Autodesk Fusion 360 part; units mm, degrees
(part 2 of 2)
  constraint parallel L239 L241
  constraint parallel L240 L242
  constraint tangent L240 A253
  constraint tangent A253 L241
  constraint tangent A254 L242
  constraint tangent L241 A254
  constraint tangent L237 A250
  constraint tangent A250 L238
  constraint tangent L238 A251
  constraint tangent L242 A255
  constraint tangent L239 A255
  constraint tangent L239 A252
  constraint tangent A252 L240
  constraint horizontal L243
  constraint perpendicular L243 L244
  constraint parallel L243 L245
  constraint parallel L244 L246
  constraint tangent A259 L246
  constraint tangent L245 A259
  constraint tangent L244 A258
  constraint tangent A258 L245
  constraint tangent A257 L244
  constraint tangent L243 A257
  constraint tangent A256 L243
  constraint tangent A256 L246
  constraint tangent L247 A260
  constraint tangent L249 A260
  constraint tangent L248 A261
  constraint tangent L249 A261
  constraint tangent L205 A262
  constraint tangent L250 A262
  constraint tangent L206 A263
  constraint tangent L250 A263
  constraint tangent L218 A264
  constraint tangent L251 A264
  constraint tangent L219 A265
  constraint tangent L251 A265
  constraint tangent L195 A266
  constraint tangent L252 A266
  constraint tangent L194 A267
  constraint tangent L252 A267
  constraint tangent L109 A268
  measures "d1" diameter of A0
  measures "d2" diameter of A1
  measures "d3" diameter of A2
  measures "d4" diameter of A3
  measures "d5" diameter of A4
  measures "d9" diameter of A110
  measures "d12" diameter of A111
  measures "d318" diameter of A181
  measures "d319" diameter of A182
extrude "Extrude1" add sketch "mriya-bumper-mjf" along normal blind 10.5 contours L106 L107 L147 A142 L148 L164 L165 A158 | L106 L107 L138 A133 L139 A134 L140 A135 L141 A136 L142 A137 L143 A138 L144 A139 L145 A140 L146 A141 L147 L148 A143 L149 A144 L150 A145 L151 A146 L152 A147 L153 A148 L154 A149 L155 A150 L156 A151 L157 A152 L158 A153 L159 A154 L160 L161 L162 L163 L164 L165 L166 L167 L168 L169 L170 L171 L172 L173 L174 A155 A156 A157 A159 A160 A161 A162 A163 L180 L181 L182 L183 L184 L185 L186 A168 A169 A170 A171 A172 A173 A174 A175 A176 A177 A178 A179 A180 makes body 1
extrude "Extrude2" add sketch "mriya-bumper-mjf" along normal blind 17 contours L106 L107 L147 A142 L148 L164 L165 A158 bodies 1
extrude "Extrude3" add sketch "mriya-bumper-mjf" along normal blind 2 from surface at 1.7 contours L108 L109 L110 L138 A133 L139 A134 L140 A135 L141 A136 L142 A137 L143 A138 L144 A139 L145 A140 L146 A141 L147 L148 A143 L149 A144 L150 A145 L151 A146 L152 A147 L153 A148 L154 A149 L155 A150 L156 A151 L157 A152 L158 A153 L159 A154 A183 A184 A185 A186 A268 | L110 L148 A183 A184 | L108 L109 L147 A142 L148 A185 A186 A268 | A113 | A114 | A115 | A116 | A181 | A182 bodies 1
extrude "Extrude6" add sketch "mriya-bumper-mjf" along normal blind 1 from surface at 14.3 contours L108 L109 L147 A142 L148 A185 A186 A268 bodies 1
extrude "Extrude13" add sketch "mriya-bumper-mjf" along normal blind 1 from surface at 7.7 contours L110 L148 A183 A184 bodies 1
chamfer "Chamfer7" distance 0.599 angle 45 4 edges at (-7, 58.2432, 14.3) (-7.4686, 77.6246, 14.3) (-14.85, 78.0932, 14.3) (-7, 9.5932, 7.7) on bodies 1
sketch "power-switch" plane through (-4.5, 0, 0) normal (1, 0, 0) x (0, 1, 0)
  line L0 (1.9932, 0) -> (76.4932, 0)
  line L1 (76.4932, 0) -> (76.4932, 17)
  line L2 (76.4932, 17) -> (19.2932, 17)
  line L3 (19.2932, 17) -> (19.2932, 10.5)
  line L4 (19.2932, 10.5) -> (1.9932, 10.5)
  line L5 (1.9932, 10.5) -> (1.9932, 0)
  line L6 (35.9932, 5.2) -> (25.7932, 5.2)
  line L7 (25.7932, 5.2) -> (25.7932, 7.9)
  line L8 (25.7932, 7.9) -> (35.9932, 7.9)
  line L9 (35.9932, 7.9) -> (35.9932, 5.2)
  line L10 (37.3932, 2.8) -> (24.3932, 2.8)
  line L11 (23.3932, 3.8) -> (23.3932, 9.3)
  line L12 (24.3932, 10.3) -> (37.3932, 10.3)
  line L13 (38.3932, 9.3) -> (38.3932, 3.8)
  arc A0 (24.3932, 10.3) -> (23.3932, 9.3) centre (24.3932, 9.3) ccw
  arc A1 (38.3932, 9.3) -> (37.3932, 10.3) centre (37.3932, 9.3) ccw
  arc A2 (37.3932, 2.8) -> (38.3932, 3.8) centre (37.3932, 3.8) ccw
  arc A3 (23.3932, 3.8) -> (24.3932, 2.8) centre (24.3932, 3.8) ccw
  line L14 (19.2932, 10.5) -> (1.8932, 10.5)
  line L15 (1.8932, 10.5) -> (1.8932, 0)
  line L16 (1.8932, 0) -> (76.5932, 0)
  line L17 (76.5932, 0) -> (76.5932, 17)
  line L18 (76.5932, 17) -> (19.2932, 17)
  line L19 (19.2932, 17) -> (19.2932, 10.5)
  constraint perpendicular L6 L7
  constraint tangent L11 A0
  constraint tangent L12 A0
  constraint tangent L12 A1
  constraint tangent L13 A1
  constraint tangent L10 A2
  constraint tangent L13 A2
  constraint tangent L10 A3
  constraint tangent L11 A3
  constraint vertical L7
  constraint perpendicular L7 L8
  constraint vertical L9
extrude "Extrude8" cut sketch "power-switch" against normal blind 2.5 contours L6 L7 L8 L9 bodies 1
extrude "Extrude9" cut sketch "power-switch" against normal blind 1 contours L10 L11 L12 L13 A0 A1 A2 A3 bodies 1
fillet "Fillet23" radius 0.1 8 edges at (-4.5, 23.3932, 6.55) (-4.5, 23.6861, 10.0071) (-4.5, 30.8932, 10.3) (-4.5, 38.1003, 10.0071) (-4.5, 38.3932, 6.55) (-4.5, 38.1003, 3.0929) (-4.5, 30.8932, 2.8) (-4.5, 23.6861, 3.0929) on bodies 1
fillet "Fillet24" radius 1 8 edges at (-5.5, 30.8932, 2.8) (-5.5, 23.6861, 3.0929) (-5.5, 23.3932, 6.55) (-5.5, 23.6861, 10.0071) (-5.5, 30.8932, 10.3) (-5.5, 38.1003, 10.0071) (-5.5, 38.3932, 6.55) (-5.5, 38.1003, 3.0929) on bodies 1
chamfer "Chamfer4" distance 0.5 angle 45 4 edges at (-7, 30.8932, 5.2) (-7, 35.9932, 6.55) (-7, 30.8932, 7.9) (-7, 25.7932, 6.55) on bodies 1
sketch "usb-c" plane through (0, 80.5932, 0) normal (0, 1, 0) x (-1, 0, 0)
  line L0 (8.5, 0) -> (40.9017, 0)
  line L1 (40.9017, 0) -> (40.9017, 10.5)
  line L2 (40.9017, 10.5) -> (25.8, 10.5)
  line L3 (25.8, 10.5) -> (25.8, 17)
  line L4 (25.8, 17) -> (8.5, 17)
  line L5 (8.5, 17) -> (8.5, 0)
  line L6 (19.7003, 7) -> (13.1002, 7)
  line L7 (13.1002, 12.35) -> (19.7002, 12.35)
  line L8 (19.7002, 8.85) -> (13.1002, 8.85)
  line L9 (21.0002, 11.05) -> (21.0002, 10.15)
  line L10 (13.1002, 14.2) -> (19.7003, 14.2)
  line L11 (11.8003, 10.15) -> (11.8003, 11.05)
  arc A0 (13.1002, 12.35) -> (11.8003, 11.05) centre (13.1002, 11.05) ccw
  arc A1 (11.8003, 10.15) -> (13.1003, 8.85) centre (13.1002, 10.15) ccw
  arc A2 (21.0002, 11.05) -> (19.7002, 12.35) centre (19.7002, 11.05) ccw
  arc A3 (19.7002, 8.85) -> (21.0002, 10.15) centre (19.7003, 10.15) ccw
  line L12 (22.7003, 11.2) -> (22.7003, 10)
  line L13 (10.1002, 11.2) -> (10.1002, 10)
  arc A4 (22.7002, 11.2) -> (19.7003, 14.2) centre (19.7003, 11.2) ccw
  arc A5 (19.7003, 7) -> (22.7003, 10) centre (19.7003, 10) ccw
  arc A6 (13.1002, 14.2) -> (10.1002, 11.2) centre (13.1002, 11.2) ccw
  arc A7 (10.1002, 10) -> (13.1002, 7) centre (13.1002, 10) ccw
  dimension "d380" = 3
  dimension "d381" = 3
  dimension "d382" = 3
  dimension "d383" = 3
  constraint horizontal L6
  constraint tangent L11 A0
  constraint tangent L7 A0
  constraint tangent L8 A1
  constraint tangent L11 A1
  constraint tangent L7 A2
  constraint tangent L9 A2
  constraint tangent L9 A3
  constraint tangent L8 A3
  constraint parallel L11 L12
  constraint parallel L5 L13
  constraint tangent L10 A4
  constraint tangent L12 A4
  constraint tangent L12 A5
  constraint tangent L6 A5
  constraint tangent L13 A6
  constraint tangent L10 A6
  constraint tangent L6 A7
  constraint tangent L13 A7
  measures "d380" radius of A4
  measures "d381" radius of A5
  measures "d382" radius of A6
  measures "d383" radius of A7
extrude "Extrude10" cut sketch "usb-c" against normal blind 2.5 contours L7 L8 L9 L11 A0 A1 A2 A3 bodies 1
extrude "Extrude11" cut sketch "usb-c" against normal blind 1.2 contours L6 L10 L12 L13 A4 A5 A6 A7 bodies 1
fillet "Fillet16" radius 1 8 edges at (-16.4003, 79.3932, 7) (-10.9789, 79.3932, 7.8787) (-10.1003, 79.3932, 10.6) (-10.9789, 79.3932, 13.3213) (-16.4003, 79.3932, 14.2) (-21.8216, 79.3932, 13.3213) (-22.7003, 79.3932, 10.6) (-21.8216, 79.3932, 7.8787) on bodies 1
fillet "Fillet20" radius 0.1 8 edges at (-10.9789, 80.5932, 7.8787) (-10.1003, 80.5932, 10.6) (-10.9789, 80.5932, 13.3213) (-16.4003, 80.5932, 14.2) (-21.8216, 80.5932, 13.3213) (-22.7003, 80.5932, 10.6) (-21.8216, 80.5932, 7.8787) (-16.4003, 80.5932, 7) on bodies 1
fillet "Fillet27" radius 1.6 90 edges at (-4.5, 47.9432, 17) (-5.6716, 79.4216, 17) (-17.15, 80.5932, 17) (-33.3509, 80.5932, 10.5) (-41.4757, 80.7074, 10.5) (-42.3069, 81.3771, 10.5) (-43.9492, 82.5887, 10.5) (-51.5908, 82.8932, 10.5) (-58.2758, 83.0074, 10.5) (-60.2069, 84.7771, 10.5) (-62.9492, 87.0887, 10.5) (-73.4, 87.3932, 10.5) (-83.8508, 87.0887, 10.5) (-86.0931, 85.2771, 10.5) (-87.5243, 84.0074, 10.5) (-94.7092, 83.8932, 10.5) (-102.8508, 83.5887, 10.5) (-107.3431, 79.5271, 10.5) (-111.0243, 76.0074, 10.5) (-115.9592, 75.8932, 10.5) (-121.8508, 75.5887, 10.5) (-123.4931, 74.3771, 10.5) (-124.3243, 73.7074, 10.5) (-131.5491, 73.5932, 10.5) (-141.0284, 72.4216, 10.5) (-142.2, 42.8932, 10.5) (-141.0284, 13.3648, 10.5) (-120.4435, 12.1932, 10.5) (-100.9649, 12.5357, 10.5) (-96.4569, 16.5593, 10.5) (-92.76, 20.041, 10.5) (-84.5813, 20.1932, 10.5) (-75.6559, 19.7842, 10.5) (-70.5608, 11.5973, 10.5) (-65.0991, 3.0385, 10.5) (-55.9906, 2.4932, 10.5) (-48.3243, 2.379, 10.5) (-47.4931, 1.7093, 10.5) (-45.8508, 0.4977, 10.5) (-37.1092, 0.1932, 10.5) (-29.3243, 0.079, 10.5) (-28.4931, -0.5907, 10.5) (-26.8508, -1.8023, 10.5) (-16.91, -2.1068, 10.5) (-5.6716, -0.9352, 10.5) (-4.5, 10.5932, 10.5) (-24.7009, 80.5932, 0) (-5.6716, 79.4216, 0) (-4.5, 39.2432, 0) (-5.6716, -0.9352, 0) (-16.91, -2.1068, 0) (-26.8508, -1.8023, 0) (-28.4931, -0.5907, 0) (-29.3243, 0.079, 0) (-37.1092, 0.1932, 0) (-45.8508, 0.4977, 0) (-47.4931, 1.7093, 0) (-48.3243, 2.379, 0) (-55.9906, 2.4932, 0) (-65.0991, 3.0385, 0) (-70.5608, 11.5973, 0) (-75.6559, 19.7842, 0) (-84.5813, 20.1932, 0) (-92.76, 20.041, 0) (-96.4569, 16.5593, 0) (-100.9649, 12.5357, 0) (-120.4435, 12.1932, 0) (-141.0284, 13.3648, 0) (-142.2, 42.8932, 0) (-141.0284, 72.4216, 0) (-131.5491, 73.5932, 0) (-124.3243, 73.7074, 0) (-123.4931, 74.3771, 0) (-121.8508, 75.5887, 0) (-115.9592, 75.8932, 0) (-111.0243, 76.0074, 0) (-107.3431, 79.5271, 0) (-102.8508, 83.5887, 0) (-94.7092, 83.8932, 0) (-87.5243, 84.0074, 0) (-86.0931, 85.2771, 0) (-83.8508, 87.0887, 0) (-73.4, 87.3932, 0) (-62.9492, 87.0887, 0) (-60.2069, 84.7771, 0) (-58.2758, 83.0074, 0) (-51.5908, 82.8932, 0) (-43.9492, 82.5887, 0) (-42.3069, 81.3771, 0) (-41.4757, 80.7074, 0) on bodies 1
fillet "Fillet30" radius 0.6 6 edges at (-4.5, 19.2932, 12.15) (-4.9686, 19.2932, 16.5314) (-6.55, 19.2932, 17) (-25.8, 80.5932, 12.15) (-25.8, 80.1246, 16.5314) (-25.8, 78.5432, 17) on bodies 1
extrude "Extrude12" cut sketch "mriya-bumper-mjf" along normal blind 1 from surface at 1.7 contours A181 | A182 bodies 1
mirror "Mirror1" about plane through (0, 0, 0) normal (1, 0, 0) of bodies 1 makes body 2
named bodies: "Left", "Right"
